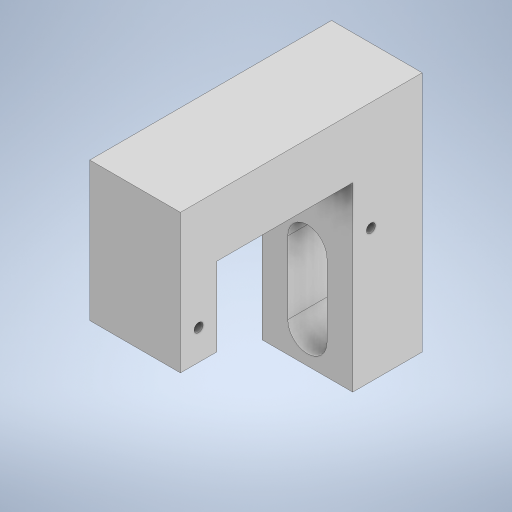
# Autodesk Inventor part: servo mount
Saved by Autodesk Inventor 2023 (Build 270158000, 158)
## iProperties
Created: 2023-03-30
Part Number: servo mount
Material: Generic
Document SubType Name: Modeling
Designer: Steven
Density: 1 g/cm^3
Appearance: Default
Author: Steven
Autodesk Inventor part; units mm, degrees
ref_plane "YZ Plane" through (0, 0, 0) normal (1, 0, 0) x (0, 1, 0)
ref_plane "XZ Plane" through (0, 0, 0) normal (0, 1, 0) x (-1, 0, 0)
ref_plane "XY Plane" through (0, 0, 0) normal (0, 0, 1) x (1, 0, 0)
sketch "Sketch1" plane through (0, 0, 0) normal (1, 0, 0) x (0, 1, 0)
  line L0 (0, 0) -> (23, 0)
  line L1 (23, 0) -> (23, -40)
  line L2 (0, 0) -> (0, -6)
  line L3 (0, -6) -> (13, -6)
  line L4 (13, -6) -> (13, -28.5)
  line L5 (13, -28.5) -> (-17, -28.5)
  line L6 (23, -40) -> (-17, -40)
  line L7 (-17, -40) -> (-17, -28.5)
  circle A0 centre (5, -3) radius 0.75
  circle A1 centre (5, -31.5) radius 0.75
  point P0 (0, -3)
  dimension "d0" = 40
  dimension "d1" = 13
  dimension "d2" = 6
  dimension "d3" = 22.5
  dimension "d4" = 1.5
  dimension "d5" = 5
  dimension "d7" = 10
  dimension "d9" = 30
  dimension "d10" = 1.5
  dimension "d11" = 3
  constraints: 17 end point, 3 horizontal, 3 vertical, 2 centre point, 2 perpendicular, 1 horizontal alignment, 1 midpoint, 1 vertical alignment
  measures "d0" distance of L0.end L1.end
  measures "d1" distance of L2.end L3.end
  measures "d2" distance of L0.start L2.end
  measures "d3" distance of L3.end L4.end
  measures "d4" diameter of A0
  measures "d5" distance from line of L2 A0.centre
  measures "d7" distance between parallel lines of L4 L1
  measures "d9" distance of L4.end L5.end
  measures "d10" diameter of A1
  measures "d11" distance from line of L5 A1.centre
extrude "Extrusion1" add sketch "Sketch1" along normal blind 15
sketch "Sketch3" plane through (0, -17, -40) normal (0, 0, -1) x (-1, 0, 0)
  line L0 (-7.5, 17) -> (-7.5, 5) construction
  line L1 (-10.75, 17) -> (-10.75, 5)
  line L2 (-4.25, 5) -> (-4.25, 17)
  arc A0 (-4.25, 17) -> (-10.75, 17) centre (-7.5, 17) ccw
  arc A1 (-10.75, 5) -> (-4.25, 5) centre (-7.5, 5) ccw
  line L3 (0, 17) -> (-15, 17) construction
  point P0 (-7.5, 11)
  point P1 (-7.5, 17)
  dimension "d14" = 6.5
  dimension "d15" = 12
  constraints: 8 end point, 4 point on circle, 4 tangent, 3 midpoint, 2 centre point, 1 parallel, 1 vertical, 1 vertical alignment
  measures "d14" diameter of A1
  measures "d15" distance of L1.start L1.end
extrude "Extrusion2" cut sketch "Sketch3" against normal up to next
body "Solid1"
